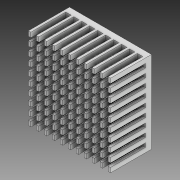
# Autodesk Inventor part: smol heatsink
Saved by Autodesk Inventor 2020 (Build 240168000, 168)
## iProperties
Created: 2020-08-04
Part Number: smol heatsink
Material: Generic
Document SubType Name: Modeling
Designer: DDeGo
Density: 1 g/cm^3
Appearance: Default
Author: DDeGo
Autodesk Inventor part; units mm, degrees
ref_plane "YZ Plane" through (0, 0, 0) normal (1, 0, 0) x (0, 1, 0)
ref_plane "XZ Plane" through (0, 0, 0) normal (0, 1, 0) x (-1, 0, 0)
ref_plane "XY Plane" through (0, 0, 0) normal (0, 0, 1) x (1, 0, 0)
sketch "Sketch1" plane through (0, 0, 0) normal (0, 0, 1) x (1, 0, 0)
  line L0 (-20, -20) -> (20, -20)
  line L1 (20, -20) -> (20, 20)
  line L2 (20, 20) -> (-20, 20)
  line L3 (-20, 20) -> (-20, -20)
  line L4 (-20, -20) -> (20, 20) construction
  line L5 (20, -20) -> (-20, 20) construction
  point P0 (0, 0)
  dimension "d0" = 40
  dimension "d1" = 40
  constraints: 12 end point, 2 midpoint, 2 parallel, 1 horizontal, 1 perpendicular
  measures "d0" distance of L1.end L2.end
  measures "d1" distance of L0.end L1.end
extrude "Extrusion1" add sketch "Sketch1" along normal blind 3
sketch "Sketch2" plane through (0, 0, 3) normal (0, 0, 1) x (1, 0, 0)
  line L0 (-20, 20) -> (-20, -20) projected
  line L1 (-20, -20) -> (-18.8, -20)
  line L2 (-18.8, -20) -> (-18.8, -17.7)
  line L3 (-18.8, -17.7) -> (-20, -17.7)
  line L4 (-20, -17.7) -> (-20, -20)
  line L5 (-20, -20) -> (20, -20) projected
  line L6 (-16.12, -20) -> (-14.92, -20)
  line L7 (-14.92, -20) -> (-14.92, -17.7)
  line L8 (-14.92, -17.7) -> (-16.12, -17.7)
  line L9 (-16.12, -17.7) -> (-16.12, -20)
  line L10 (-12.24, -20) -> (-11.04, -20)
  line L11 (-11.04, -20) -> (-11.04, -17.7)
  line L12 (-11.04, -17.7) -> (-12.24, -17.7)
  line L13 (-12.24, -17.7) -> (-12.24, -20)
  line L14 (-8.36, -20) -> (-7.16, -20)
  line L15 (-7.16, -20) -> (-7.16, -17.7)
  line L16 (-7.16, -17.7) -> (-8.36, -17.7)
  line L17 (-8.36, -17.7) -> (-8.36, -20)
  line L18 (-4.48, -20) -> (-3.28, -20)
  line L19 (-3.28, -20) -> (-3.28, -17.7)
  line L20 (-3.28, -17.7) -> (-4.48, -17.7)
  line L21 (-4.48, -17.7) -> (-4.48, -20)
  line L22 (-0.6, -20) -> (0.6, -20)
  line L23 (0.6, -20) -> (0.6, -17.7)
  line L24 (0.6, -17.7) -> (-0.6, -17.7)
  line L25 (-0.6, -17.7) -> (-0.6, -20)
  line L26 (3.28, -20) -> (4.48, -20)
  line L27 (4.48, -20) -> (4.48, -17.7)
  line L28 (4.48, -17.7) -> (3.28, -17.7)
  line L29 (3.28, -17.7) -> (3.28, -20)
  line L30 (7.16, -20) -> (8.36, -20)
  line L31 (8.36, -20) -> (8.36, -17.7)
  line L32 (8.36, -17.7) -> (7.16, -17.7)
  line L33 (7.16, -17.7) -> (7.16, -20)
  line L34 (11.04, -20) -> (12.24, -20)
  line L35 (12.24, -20) -> (12.24, -17.7)
  line L36 (12.24, -17.7) -> (11.04, -17.7)
  line L37 (11.04, -17.7) -> (11.04, -20)
  line L38 (14.92, -20) -> (16.12, -20)
  line L39 (16.12, -20) -> (16.12, -17.7)
  line L40 (16.12, -17.7) -> (14.92, -17.7)
  line L41 (14.92, -17.7) -> (14.92, -20)
  line L42 (18.8, -20) -> (20, -20)
  line L43 (20, -20) -> (20, -17.7)
  line L44 (20, -17.7) -> (18.8, -17.7)
  line L45 (18.8, -17.7) -> (18.8, -20)
  line L46 (-20, -15.8111) -> (-18.8, -15.8111)
  line L47 (-18.8, -15.8111) -> (-18.8, -13.5111)
  line L48 (-18.8, -13.5111) -> (-20, -13.5111)
  line L49 (-20, -13.5111) -> (-20, -15.8111)
  line L50 (-16.12, -15.8111) -> (-14.92, -15.8111)
  line L51 (-14.92, -15.8111) -> (-14.92, -13.5111)
  line L52 (-14.92, -13.5111) -> (-16.12, -13.5111)
  line L53 (-16.12, -13.5111) -> (-16.12, -15.8111)
  line L54 (-12.24, -15.8111) -> (-11.04, -15.8111)
  line L55 (-11.04, -15.8111) -> (-11.04, -13.5111)
  line L56 (-11.04, -13.5111) -> (-12.24, -13.5111)
  line L57 (-12.24, -13.5111) -> (-12.24, -15.8111)
  line L58 (-8.36, -15.8111) -> (-7.16, -15.8111)
  line L59 (-7.16, -15.8111) -> (-7.16, -13.5111)
  line L60 (-7.16, -13.5111) -> (-8.36, -13.5111)
  line L61 (-8.36, -13.5111) -> (-8.36, -15.8111)
  line L62 (-4.48, -15.8111) -> (-3.28, -15.8111)
  line L63 (-3.28, -15.8111) -> (-3.28, -13.5111)
  line L64 (-3.28, -13.5111) -> (-4.48, -13.5111)
  line L65 (-4.48, -13.5111) -> (-4.48, -15.8111)
  line L66 (-0.6, -15.8111) -> (0.6, -15.8111)
  line L67 (0.6, -15.8111) -> (0.6, -13.5111)
  line L68 (0.6, -13.5111) -> (-0.6, -13.5111)
  line L69 (-0.6, -13.5111) -> (-0.6, -15.8111)
  line L70 (3.28, -15.8111) -> (4.48, -15.8111)
  line L71 (4.48, -15.8111) -> (4.48, -13.5111)
  line L72 (4.48, -13.5111) -> (3.28, -13.5111)
  line L73 (3.28, -13.5111) -> (3.28, -15.8111)
  line L74 (7.16, -15.8111) -> (8.36, -15.8111)
  line L75 (8.36, -15.8111) -> (8.36, -13.5111)
  line L76 (8.36, -13.5111) -> (7.16, -13.5111)
  line L77 (7.16, -13.5111) -> (7.16, -15.8111)
  line L78 (11.04, -15.8111) -> (12.24, -15.8111)
  line L79 (12.24, -15.8111) -> (12.24, -13.5111)
  line L80 (12.24, -13.5111) -> (11.04, -13.5111)
  line L81 (11.04, -13.5111) -> (11.04, -15.8111)
  line L82 (14.92, -15.8111) -> (16.12, -15.8111)
  line L83 (16.12, -15.8111) -> (16.12, -13.5111)
  line L84 (16.12, -13.5111) -> (14.92, -13.5111)
  line L85 (14.92, -13.5111) -> (14.92, -15.8111)
  line L86 (18.8, -15.8111) -> (20, -15.8111)
  line L87 (20, -15.8111) -> (20, -13.5111)
  line L88 (20, -13.5111) -> (18.8, -13.5111)
  line L89 (18.8, -13.5111) -> (18.8, -15.8111)
  line L90 (-20, -11.6222) -> (-18.8, -11.6222)
  line L91 (-18.8, -11.6222) -> (-18.8, -9.3222)
  line L92 (-18.8, -9.3222) -> (-20, -9.3222)
  line L93 (-20, -9.3222) -> (-20, -11.6222)
  line L94 (-16.12, -11.6222) -> (-14.92, -11.6222)
  line L95 (-14.92, -11.6222) -> (-14.92, -9.3222)
  line L96 (-14.92, -9.3222) -> (-16.12, -9.3222)
  line L97 (-16.12, -9.3222) -> (-16.12, -11.6222)
  line L98 (-12.24, -11.6222) -> (-11.04, -11.6222)
  line L99 (-11.04, -11.6222) -> (-11.04, -9.3222)
  line L100 (-11.04, -9.3222) -> (-12.24, -9.3222)
  line L101 (-12.24, -9.3222) -> (-12.24, -11.6222)
  line L102 (-8.36, -11.6222) -> (-7.16, -11.6222)
  line L103 (-7.16, -11.6222) -> (-7.16, -9.3222)
  line L104 (-7.16, -9.3222) -> (-8.36, -9.3222)
  line L105 (-8.36, -9.3222) -> (-8.36, -11.6222)
  line L106 (-4.48, -11.6222) -> (-3.28, -11.6222)
  line L107 (-3.28, -11.6222) -> (-3.28, -9.3222)
  line L108 (-3.28, -9.3222) -> (-4.48, -9.3222)
  line L109 (-4.48, -9.3222) -> (-4.48, -11.6222)
  line L110 (-0.6, -11.6222) -> (0.6, -11.6222)
  line L111 (0.6, -11.6222) -> (0.6, -9.3222)
  line L112 (0.6, -9.3222) -> (-0.6, -9.3222)
  line L113 (-0.6, -9.3222) -> (-0.6, -11.6222)
  line L114 (3.28, -11.6222) -> (4.48, -11.6222)
  line L115 (4.48, -11.6222) -> (4.48, -9.3222)
  line L116 (4.48, -9.3222) -> (3.28, -9.3222)
  line L117 (3.28, -9.3222) -> (3.28, -11.6222)
  line L118 (7.16, -11.6222) -> (8.36, -11.6222)
  line L119 (8.36, -11.6222) -> (8.36, -9.3222)
  line L120 (8.36, -9.3222) -> (7.16, -9.3222)
  line L121 (7.16, -9.3222) -> (7.16, -11.6222)
  line L122 (11.04, -11.6222) -> (12.24, -11.6222)
  line L123 (12.24, -11.6222) -> (12.24, -9.3222)
  line L124 (12.24, -9.3222) -> (11.04, -9.3222)
  line L125 (11.04, -9.3222) -> (11.04, -11.6222)
  line L126 (14.92, -11.6222) -> (16.12, -11.6222)
  line L127 (16.12, -11.6222) -> (16.12, -9.3222)
  line L128 (16.12, -9.3222) -> (14.92, -9.3222)
  line L129 (14.92, -9.3222) -> (14.92, -11.6222)
  line L130 (18.8, -11.6222) -> (20, -11.6222)
  line L131 (20, -11.6222) -> (20, -9.3222)
  line L132 (20, -9.3222) -> (18.8, -9.3222)
  line L133 (18.8, -9.3222) -> (18.8, -11.6222)
  line L134 (-20, -7.4333) -> (-18.8, -7.4333)
  line L135 (-18.8, -7.4333) -> (-18.8, -5.1333)
  line L136 (-18.8, -5.1333) -> (-20, -5.1333)
  line L137 (-20, -5.1333) -> (-20, -7.4333)
  line L138 (-16.12, -7.4333) -> (-14.92, -7.4333)
  line L139 (-14.92, -7.4333) -> (-14.92, -5.1333)
  line L140 (-14.92, -5.1333) -> (-16.12, -5.1333)
  line L141 (-16.12, -5.1333) -> (-16.12, -7.4333)
  line L142 (-12.24, -7.4333) -> (-11.04, -7.4333)
  line L143 (-11.04, -7.4333) -> (-11.04, -5.1333)
  line L144 (-11.04, -5.1333) -> (-12.24, -5.1333)
  line L145 (-12.24, -5.1333) -> (-12.24, -7.4333)
  line L146 (-8.36, -7.4333) -> (-7.16, -7.4333)
  line L147 (-7.16, -7.4333) -> (-7.16, -5.1333)
  line L148 (-7.16, -5.1333) -> (-8.36, -5.1333)
  line L149 (-8.36, -5.1333) -> (-8.36, -7.4333)
  line L150 (-4.48, -7.4333) -> (-3.28, -7.4333)
  line L151 (-3.28, -7.4333) -> (-3.28, -5.1333)
  line L152 (-3.28, -5.1333) -> (-4.48, -5.1333)
  line L153 (-4.48, -5.1333) -> (-4.48, -7.4333)
  line L154 (-0.6, -7.4333) -> (0.6, -7.4333)
  line L155 (0.6, -7.4333) -> (0.6, -5.1333)
  line L156 (0.6, -5.1333) -> (-0.6, -5.1333)
  line L157 (-0.6, -5.1333) -> (-0.6, -7.4333)
  line L158 (3.28, -7.4333) -> (4.48, -7.4333)
  line L159 (4.48, -7.4333) -> (4.48, -5.1333)
  line L160 (4.48, -5.1333) -> (3.28, -5.1333)
  line L161 (3.28, -5.1333) -> (3.28, -7.4333)
  line L162 (7.16, -7.4333) -> (8.36, -7.4333)
  line L163 (8.36, -7.4333) -> (8.36, -5.1333)
  line L164 (8.36, -5.1333) -> (7.16, -5.1333)
  line L165 (7.16, -5.1333) -> (7.16, -7.4333)
  line L166 (11.04, -7.4333) -> (12.24, -7.4333)
  line L167 (12.24, -7.4333) -> (12.24, -5.1333)
  line L168 (12.24, -5.1333) -> (11.04, -5.1333)
  line L169 (11.04, -5.1333) -> (11.04, -7.4333)
  line L170 (14.92, -7.4333) -> (16.12, -7.4333)
  line L171 (16.12, -7.4333) -> (16.12, -5.1333)
  line L172 (16.12, -5.1333) -> (14.92, -5.1333)
  line L173 (14.92, -5.1333) -> (14.92, -7.4333)
  line L174 (18.8, -7.4333) -> (20, -7.4333)
  line L175 (20, -7.4333) -> (20, -5.1333)
  line L176 (20, -5.1333) -> (18.8, -5.1333)
  line L177 (18.8, -5.1333) -> (18.8, -7.4333)
  line L178 (-20, -3.2444) -> (-18.8, -3.2444)
  line L179 (-18.8, -3.2444) -> (-18.8, -0.9444)
  line L180 (-18.8, -0.9444) -> (-20, -0.9444)
  line L181 (-20, -0.9444) -> (-20, -3.2444)
  line L182 (-16.12, -3.2444) -> (-14.92, -3.2444)
  line L183 (-14.92, -3.2444) -> (-14.92, -0.9444)
  line L184 (-14.92, -0.9444) -> (-16.12, -0.9444)
  line L185 (-16.12, -0.9444) -> (-16.12, -3.2444)
  line L186 (-12.24, -3.2444) -> (-11.04, -3.2444)
  line L187 (-11.04, -3.2444) -> (-11.04, -0.9444)
  line L188 (-11.04, -0.9444) -> (-12.24, -0.9444)
  line L189 (-12.24, -0.9444) -> (-12.24, -3.2444)
  line L190 (-8.36, -3.2444) -> (-7.16, -3.2444)
  line L191 (-7.16, -3.2444) -> (-7.16, -0.9444)
  line L192 (-7.16, -0.9444) -> (-8.36, -0.9444)
  line L193 (-8.36, -0.9444) -> (-8.36, -3.2444)
  line L194 (-4.48, -3.2444) -> (-3.28, -3.2444)
  line L195 (-3.28, -3.2444) -> (-3.28, -0.9444)
  line L196 (-3.28, -0.9444) -> (-4.48, -0.9444)
  line L197 (-4.48, -0.9444) -> (-4.48, -3.2444)
  line L198 (-0.6, -3.2444) -> (0.6, -3.2444)
  line L199 (0.6, -3.2444) -> (0.6, -0.9444)
  line L200 (0.6, -0.9444) -> (-0.6, -0.9444)
  line L201 (-0.6, -0.9444) -> (-0.6, -3.2444)
  line L202 (3.28, -3.2444) -> (4.48, -3.2444)
  line L203 (4.48, -3.2444) -> (4.48, -0.9444)
  line L204 (4.48, -0.9444) -> (3.28, -0.9444)
  line L205 (3.28, -0.9444) -> (3.28, -3.2444)
  line L206 (7.16, -3.2444) -> (8.36, -3.2444)
  line L207 (8.36, -3.2444) -> (8.36, -0.9444)
  line L208 (8.36, -0.9444) -> (7.16, -0.9444)
  line L209 (7.16, -0.9444) -> (7.16, -3.2444)
  line L210 (11.04, -3.2444) -> (12.24, -3.2444)
  line L211 (12.24, -3.2444) -> (12.24, -0.9444)
  line L212 (12.24, -0.9444) -> (11.04, -0.9444)
  line L213 (11.04, -0.9444) -> (11.04, -3.2444)
  line L214 (14.92, -3.2444) -> (16.12, -3.2444)
  line L215 (16.12, -3.2444) -> (16.12, -0.9444)
  line L216 (16.12, -0.9444) -> (14.92, -0.9444)
  line L217 (14.92, -0.9444) -> (14.92, -3.2444)
  line L218 (18.8, -3.2444) -> (20, -3.2444)
  line L219 (20, -3.2444) -> (20, -0.9444)
  line L220 (20, -0.9444) -> (18.8, -0.9444)
  line L221 (18.8, -0.9444) -> (18.8, -3.2444)
  line L222 (-20, 0.9444) -> (-18.8, 0.9444)
  line L223 (-18.8, 0.9444) -> (-18.8, 3.2444)
  line L224 (-18.8, 3.2444) -> (-20, 3.2444)
  line L225 (-20, 3.2444) -> (-20, 0.9444)
  line L226 (-16.12, 0.9444) -> (-14.92, 0.9444)
  line L227 (-14.92, 0.9444) -> (-14.92, 3.2444)
  line L228 (-14.92, 3.2444) -> (-16.12, 3.2444)
  line L229 (-16.12, 3.2444) -> (-16.12, 0.9444)
  line L230 (-12.24, 0.9444) -> (-11.04, 0.9444)
  line L231 (-11.04, 0.9444) -> (-11.04, 3.2444)
  line L232 (-11.04, 3.2444) -> (-12.24, 3.2444)
  line L233 (-12.24, 3.2444) -> (-12.24, 0.9444)
  line L234 (-8.36, 0.9444) -> (-7.16, 0.9444)
  line L235 (-7.16, 0.9444) -> (-7.16, 3.2444)
  line L236 (-7.16, 3.2444) -> (-8.36, 3.2444)
  line L237 (-8.36, 3.2444) -> (-8.36, 0.9444)
  line L238 (-4.48, 0.9444) -> (-3.28, 0.9444)
  line L239 (-3.28, 0.9444) -> (-3.28, 3.2444)
  line L240 (-3.28, 3.2444) -> (-4.48, 3.2444)
  line L241 (-4.48, 3.2444) -> (-4.48, 0.9444)
  line L242 (-0.6, 0.9444) -> (0.6, 0.9444)
  line L243 (0.6, 0.9444) -> (0.6, 3.2444)
  line L244 (0.6, 3.2444) -> (-0.6, 3.2444)
  line L245 (-0.6, 3.2444) -> (-0.6, 0.9444)
  line L246 (3.28, 0.9444) -> (4.48, 0.9444)
  line L247 (4.48, 0.9444) -> (4.48, 3.2444)
  line L248 (4.48, 3.2444) -> (3.28, 3.2444)
  line L249 (3.28, 3.2444) -> (3.28, 0.9444)
  line L250 (7.16, 0.9444) -> (8.36, 0.9444)
  line L251 (8.36, 0.9444) -> (8.36, 3.2444)
  line L252 (8.36, 3.2444) -> (7.16, 3.2444)
  line L253 (7.16, 3.2444) -> (7.16, 0.9444)
  line L254 (11.04, 0.9444) -> (12.24, 0.9444)
  line L255 (12.24, 0.9444) -> (12.24, 3.2444)
  line L256 (12.24, 3.2444) -> (11.04, 3.2444)
  line L257 (11.04, 3.2444) -> (11.04, 0.9444)
  line L258 (14.92, 0.9444) -> (16.12, 0.9444)
  line L259 (16.12, 0.9444) -> (16.12, 3.2444)
  line L260 (16.12, 3.2444) -> (14.92, 3.2444)
  line L261 (14.92, 3.2444) -> (14.92, 0.9444)
  line L262 (18.8, 0.9444) -> (20, 0.9444)
  line L263 (20, 0.9444) -> (20, 3.2444)
  line L264 (20, 3.2444) -> (18.8, 3.2444)
  line L265 (18.8, 3.2444) -> (18.8, 0.9444)
  line L266 (-20, 5.1333) -> (-18.8, 5.1333)
  line L267 (-18.8, 5.1333) -> (-18.8, 7.4333)
  line L268 (-18.8, 7.4333) -> (-20, 7.4333)
  line L269 (-20, 7.4333) -> (-20, 5.1333)
  line L270 (-16.12, 5.1333) -> (-14.92, 5.1333)
  line L271 (-14.92, 5.1333) -> (-14.92, 7.4333)
  line L272 (-14.92, 7.4333) -> (-16.12, 7.4333)
  line L273 (-16.12, 7.4333) -> (-16.12, 5.1333)
  line L274 (-12.24, 5.1333) -> (-11.04, 5.1333)
  line L275 (-11.04, 5.1333) -> (-11.04, 7.4333)
  line L276 (-11.04, 7.4333) -> (-12.24, 7.4333)
  line L277 (-12.24, 7.4333) -> (-12.24, 5.1333)
  line L278 (-8.36, 5.1333) -> (-7.16, 5.1333)
  line L279 (-7.16, 5.1333) -> (-7.16, 7.4333)
  line L280 (-7.16, 7.4333) -> (-8.36, 7.4333)
  line L281 (-8.36, 7.4333) -> (-8.36, 5.1333)
  line L282 (-4.48, 5.1333) -> (-3.28, 5.1333)
  line L283 (-3.28, 5.1333) -> (-3.28, 7.4333)
  line L284 (-3.28, 7.4333) -> (-4.48, 7.4333)
  line L285 (-4.48, 7.4333) -> (-4.48, 5.1333)
  line L286 (-0.6, 5.1333) -> (0.6, 5.1333)
  line L287 (0.6, 5.1333) -> (0.6, 7.4333)
  line L288 (0.6, 7.4333) -> (-0.6, 7.4333)
  line L289 (-0.6, 7.4333) -> (-0.6, 5.1333)
  line L290 (3.28, 5.1333) -> (4.48, 5.1333)
  line L291 (4.48, 5.1333) -> (4.48, 7.4333)
  line L292 (4.48, 7.4333) -> (3.28, 7.4333)
  line L293 (3.28, 7.4333) -> (3.28, 5.1333)
  line L294 (7.16, 5.1333) -> (8.36, 5.1333)
  line L295 (8.36, 5.1333) -> (8.36, 7.4333)
  line L296 (8.36, 7.4333) -> (7.16, 7.4333)
  line L297 (7.16, 7.4333) -> (7.16, 5.1333)
  line L298 (11.04, 5.1333) -> (12.24, 5.1333)
  line L299 (12.24, 5.1333) -> (12.24, 7.4333)
  line L300 (12.24, 7.4333) -> (11.04, 7.4333)
  line L301 (11.04, 7.4333) -> (11.04, 5.1333)
  line L302 (14.92, 5.1333) -> (16.12, 5.1333)
  line L303 (16.12, 5.1333) -> (16.12, 7.4333)
  line L304 (16.12, 7.4333) -> (14.92, 7.4333)
  line L305 (14.92, 7.4333) -> (14.92, 5.1333)
  line L306 (18.8, 5.1333) -> (20, 5.1333)
  line L307 (20, 5.1333) -> (20, 7.4333)
  line L308 (20, 7.4333) -> (18.8, 7.4333)
  line L309 (18.8, 7.4333) -> (18.8, 5.1333)
  line L310 (-20, 9.3222) -> (-18.8, 9.3222)
  line L311 (-18.8, 9.3222) -> (-18.8, 11.6222)
  line L312 (-18.8, 11.6222) -> (-20, 11.6222)
  line L313 (-20, 11.6222) -> (-20, 9.3222)
  line L314 (-16.12, 9.3222) -> (-14.92, 9.3222)
  line L315 (-14.92, 9.3222) -> (-14.92, 11.6222)
  line L316 (-14.92, 11.6222) -> (-16.12, 11.6222)
  line L317 (-16.12, 11.6222) -> (-16.12, 9.3222)
  line L318 (-12.24, 9.3222) -> (-11.04, 9.3222)
  line L319 (-11.04, 9.3222) -> (-11.04, 11.6222)
  line L320 (-11.04, 11.6222) -> (-12.24, 11.6222)
  line L321 (-12.24, 11.6222) -> (-12.24, 9.3222)
  line L322 (-8.36, 9.3222) -> (-7.16, 9.3222)
  line L323 (-7.16, 9.3222) -> (-7.16, 11.6222)
  line L324 (-7.16, 11.6222) -> (-8.36, 11.6222)
  line L325 (-8.36, 11.6222) -> (-8.36, 9.3222)
  line L326 (-4.48, 9.3222) -> (-3.28, 9.3222)
  line L327 (-3.28, 9.3222) -> (-3.28, 11.6222)
  line L328 (-3.28, 11.6222) -> (-4.48, 11.6222)
  line L329 (-4.48, 11.6222) -> (-4.48, 9.3222)
  line L330 (-0.6, 9.3222) -> (0.6, 9.3222)
  line L331 (0.6, 9.3222) -> (0.6, 11.6222)
  line L332 (0.6, 11.6222) -> (-0.6, 11.6222)
  line L333 (-0.6, 11.6222) -> (-0.6, 9.3222)
  line L334 (3.28, 9.3222) -> (4.48, 9.3222)
  line L335 (4.48, 9.3222) -> (4.48, 11.6222)
  line L336 (4.48, 11.6222) -> (3.28, 11.6222)
  line L337 (3.28, 11.6222) -> (3.28, 9.3222)
  line L338 (7.16, 9.3222) -> (8.36, 9.3222)
  line L339 (8.36, 9.3222) -> (8.36, 11.6222)
  line L340 (8.36, 11.6222) -> (7.16, 11.6222)
  line L341 (7.16, 11.6222) -> (7.16, 9.3222)
  line L342 (11.04, 9.3222) -> (12.24, 9.3222)
  line L343 (12.24, 9.3222) -> (12.24, 11.6222)
  line L344 (12.24, 11.6222) -> (11.04, 11.6222)
  line L345 (11.04, 11.6222) -> (11.04, 9.3222)
  line L346 (14.92, 9.3222) -> (16.12, 9.3222)
  line L347 (16.12, 9.3222) -> (16.12, 11.6222)
  line L348 (16.12, 11.6222) -> (14.92, 11.6222)
  line L349 (14.92, 11.6222) -> (14.92, 9.3222)
  line L350 (18.8, 9.3222) -> (20, 9.3222)
  line L351 (20, 9.3222) -> (20, 11.6222)
  line L352 (20, 11.6222) -> (18.8, 11.6222)
  line L353 (18.8, 11.6222) -> (18.8, 9.3222)
  line L354 (-20, 13.5111) -> (-18.8, 13.5111)
  line L355 (-18.8, 13.5111) -> (-18.8, 15.8111)
  line L356 (-18.8, 15.8111) -> (-20, 15.8111)
  line L357 (-20, 15.8111) -> (-20, 13.5111)
  line L358 (-16.12, 13.5111) -> (-14.92, 13.5111)
  line L359 (-14.92, 13.5111) -> (-14.92, 15.8111)
  line L360 (-14.92, 15.8111) -> (-16.12, 15.8111)
  line L361 (-16.12, 15.8111) -> (-16.12, 13.5111)
  line L362 (-12.24, 13.5111) -> (-11.04, 13.5111)
  line L363 (-11.04, 13.5111) -> (-11.04, 15.8111)
  line L364 (-11.04, 15.8111) -> (-12.24, 15.8111)
  line L365 (-12.24, 15.8111) -> (-12.24, 13.5111)
  line L366 (-8.36, 13.5111) -> (-7.16, 13.5111)
  line L367 (-7.16, 13.5111) -> (-7.16, 15.8111)
  line L368 (-7.16, 15.8111) -> (-8.36, 15.8111)
  line L369 (-8.36, 15.8111) -> (-8.36, 13.5111)
  line L370 (-4.48, 13.5111) -> (-3.28, 13.5111)
  line L371 (-3.28, 13.5111) -> (-3.28, 15.8111)
  line L372 (-3.28, 15.8111) -> (-4.48, 15.8111)
  line L373 (-4.48, 15.8111) -> (-4.48, 13.5111)
  line L374 (-0.6, 13.5111) -> (0.6, 13.5111)
  line L375 (0.6, 13.5111) -> (0.6, 15.8111)
  line L376 (0.6, 15.8111) -> (-0.6, 15.8111)
  line L377 (-0.6, 15.8111) -> (-0.6, 13.5111)
  line L378 (3.28, 13.5111) -> (4.48, 13.5111)
  line L379 (4.48, 13.5111) -> (4.48, 15.8111)
  line L380 (4.48, 15.8111) -> (3.28, 15.8111)
  line L381 (3.28, 15.8111) -> (3.28, 13.5111)
  line L382 (7.16, 13.5111) -> (8.36, 13.5111)
  line L383 (8.36, 13.5111) -> (8.36, 15.8111)
  line L384 (8.36, 15.8111) -> (7.16, 15.8111)
  line L385 (7.16, 15.8111) -> (7.16, 13.5111)
  line L386 (11.04, 13.5111) -> (12.24, 13.5111)
  line L387 (12.24, 13.5111) -> (12.24, 15.8111)
  line L388 (12.24, 15.8111) -> (11.04, 15.8111)
  line L389 (11.04, 15.8111) -> (11.04, 13.5111)
  line L390 (14.92, 13.5111) -> (16.12, 13.5111)
  line L391 (16.12, 13.5111) -> (16.12, 15.8111)
  line L392 (16.12, 15.8111) -> (14.92, 15.8111)
  line L393 (14.92, 15.8111) -> (14.92, 13.5111)
  line L394 (18.8, 13.5111) -> (20, 13.5111)
  line L395 (20, 13.5111) -> (20, 15.8111)
  line L396 (20, 15.8111) -> (18.8, 15.8111)
  line L397 (18.8, 15.8111) -> (18.8, 13.5111)
  line L398 (-20, 17.7) -> (-18.8, 17.7)
  line L399 (-18.8, 17.7) -> (-18.8, 20)
  line L400 (-18.8, 20) -> (-20, 20)
  line L401 (-20, 20) -> (-20, 17.7)
  line L402 (-16.12, 17.7) -> (-14.92, 17.7)
  line L403 (-14.92, 17.7) -> (-14.92, 20)
  line L404 (-14.92, 20) -> (-16.12, 20)
  line L405 (-16.12, 20) -> (-16.12, 17.7)
  line L406 (-12.24, 17.7) -> (-11.04, 17.7)
  line L407 (-11.04, 17.7) -> (-11.04, 20)
  line L408 (-11.04, 20) -> (-12.24, 20)
  line L409 (-12.24, 20) -> (-12.24, 17.7)
  line L410 (-8.36, 17.7) -> (-7.16, 17.7)
  line L411 (-7.16, 17.7) -> (-7.16, 20)
  line L412 (-7.16, 20) -> (-8.36, 20)
  line L413 (-8.36, 20) -> (-8.36, 17.7)
  line L414 (-4.48, 17.7) -> (-3.28, 17.7)
  line L415 (-3.28, 17.7) -> (-3.28, 20)
  line L416 (-3.28, 20) -> (-4.48, 20)
  line L417 (-4.48, 20) -> (-4.48, 17.7)
  line L418 (-0.6, 17.7) -> (0.6, 17.7)
  line L419 (0.6, 17.7) -> (0.6, 20)
  line L420 (0.6, 20) -> (-0.6, 20)
  line L421 (-0.6, 20) -> (-0.6, 17.7)
  line L422 (3.28, 17.7) -> (4.48, 17.7)
  line L423 (4.48, 17.7) -> (4.48, 20)
  line L424 (4.48, 20) -> (3.28, 20)
  line L425 (3.28, 20) -> (3.28, 17.7)
  line L426 (7.16, 17.7) -> (8.36, 17.7)
  line L427 (8.36, 17.7) -> (8.36, 20)
  line L428 (8.36, 20) -> (7.16, 20)
  line L429 (7.16, 20) -> (7.16, 17.7)
  line L430 (11.04, 17.7) -> (12.24, 17.7)
  line L431 (12.24, 17.7) -> (12.24, 20)
  line L432 (12.24, 20) -> (11.04, 20)
  line L433 (11.04, 20) -> (11.04, 17.7)
  line L434 (14.92, 17.7) -> (16.12, 17.7)
  line L435 (16.12, 17.7) -> (16.12, 20)
  line L436 (16.12, 20) -> (14.92, 20)
  line L437 (14.92, 20) -> (14.92, 17.7)
  line L438 (18.8, 17.7) -> (20, 17.7)
  line L439 (20, 17.7) -> (20, 20)
  line L440 (20, 20) -> (18.8, 20)
  line L441 (18.8, 20) -> (18.8, 17.7)
  line L442 (20, 20) -> (-20, 20) projected
  line L443 (20, -20) -> (20, 20) projected
  point P0 (0, 0)
  point P1 (20, -20)
  dimension "d4" = 2.3
  dimension "d5" = 1.2
  dimension "d8" = 3.88
  dimension "d11" = 4.1889
  constraints: 880 end point, 40 horizontal alignment, 22 parallel, 20 collinear, 1 coincident, 1 horizontal, 1 perpendicular, 1 vertical, 793 other
  measures "d4" distance of L1.end L2.end
  measures "d5" distance of L2.end L3.end
  measures "d8" distance of L0.end L6.start
  measures "d11" distance of L0.end L46.start
extrude "Extrusion2" add sketch "Sketch2" along normal blind 17 contours L400 L399 L398 L0 | L356 L355 L354 L0 | L404 L403 L402 L405 | L312 L311 L310 L0 | L408 L407 L406 L409 | L268 L267 L266 L0 | L412 L411 L410 L413 | L224 L223 L222 L0 | L416 L415 L414 L417 | L180 L179 L178 L0 | L420 L419 L418 L421 | L136 L135 L134 L0 | L424 L423 L422 L425 | L92 L91 L90 L0 | L428 L427 L426 L429 | L48 L47 L46 L0 | L432 L431 L430 L433 | L3 L2 L1 L0 | L436 L435 L434 L437 | L440 L439 L438 L441 | L9 L8 L7 L5 | L13 L12 L11 L5 | L395 L394 L397 L396 | L17 L16 L15 L5 | L351 L350 L353 L352 | L21 L20 L19 L5 | L307 L306 L309 L308 | L25 L24 L23 L5 | L263 L262 L265 L264 | L29 L28 L27 L5 | L219 L218 L221 L220 | L33 L32 L31 L5 | L175 L174 L177 L176 | L37 L36 L35 L5 | L131 L130 L133 L132 | L41 L40 L39 L5 | L87 L86 L89 L88 | L45 L44 L43 L5 | L53 L52 L51 L50 | L57 L56 L55 L54 | L61 L60 L59 L58 | L65 L64 L63 L62 | L69 L68 L67 L66 | L73 L72 L71 L70 | L77 L76 L75 L74 | L81 L80 L79 L78 | L85 L84 L83 L82 | L97 L96 L95 L94 | L101 L100 L99 L98 | L105 L104 L103 L102 | L109 L108 L107 L106 | L113 L112 L111 L110 | L117 L116 L115 L114 | L121 L120 L119 L118 | L125 L124 L123 L122 | L129 L128 L127 L126 | L141 L140 L139 L138 | L145 L144 L143 L142 | L149 L148 L147 L146 | L153 L152 L151 L150 | L157 L156 L155 L154 | L161 L160 L159 L158 | L165 L164 L163 L162 | L169 L168 L167 L166 | L173 L172 L171 L170 | L185 L184 L183 L182 | L189 L188 L187 L186 | L193 L192 L191 L190 | L197 L196 L195 L194 | L201 L200 L199 L198 | L205 L204 L203 L202 | L209 L208 L207 L206 | L213 L212 L211 L210 | L217 L216 L215 L214 | L229 L228 L227 L226 | L233 L232 L231 L230 | L237 L236 L235 L234 | L241 L240 L239 L238 | L245 L244 L243 L242 | L249 L248 L247 L246 | L253 L252 L251 L250 | L257 L256 L255 L254 | L261 L260 L259 L258 | L273 L272 L271 L270 | L277 L276 L275 L274 | L281 L280 L279 L278 | L285 L284 L283 L282 | L289 L288 L287 L286 | L293 L292 L291 L290 | L297 L296 L295 L294 | L301 L300 L299 L298 | L305 L304 L303 L302 | L317 L316 L315 L314 | L321 L320 L319 L318 | L325 L324 L323 L322 | L329 L328 L327 L326 | L333 L332 L331 L330 | L337 L336 L335 L334 | L341 L340 L339 L338 | L345 L344 L343 L342 | L349 L348 L347 L346 | L361 L360 L359 L358 | L365 L364 L363 L362 | L369 L368 L367 L366 | L373 L372 L371 L370 | L377 L376 L375 L374 | L381 L380 L379 L378 | L385 L384 L383 L382 | L389 L388 L387 L386 | L393 L392 L391 L390
body "Solid1"
